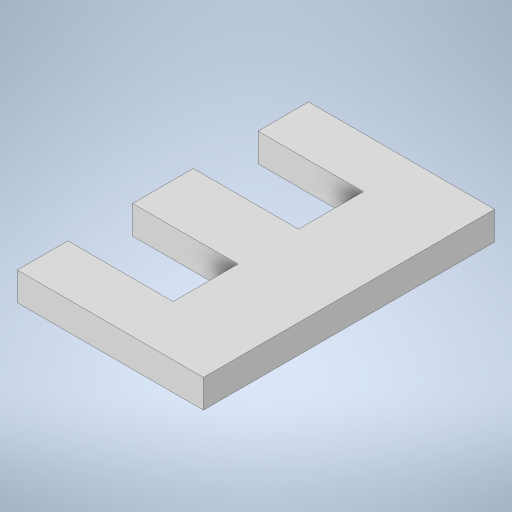
# Autodesk Inventor part: base
Saved by Autodesk Inventor 2024.3 (Build 283343000, 343)
## iProperties
Created: 2024-10-09
Part Number: base
Material: Generic
Document SubType Name: Modeling
Designer: pjcaa
Density: 1 g/cm^3
Appearance: Default
Author: pjcaa
Autodesk Inventor part; units mm, degrees
ref_plane "YZ Plane" through (0, 0, 0) normal (1, 0, 0) x (0, 1, 0)
ref_plane "XZ Plane" through (0, 0, 0) normal (0, 1, 0) x (-1, 0, 0)
ref_plane "XY Plane" through (0, 0, 0) normal (0, 0, 1) x (1, 0, 0)
sketch "Sketch16" plane through (0, 0, 0) normal (0, 0, 1) x (1, 0, 0)
  line L0 (-9, 5.75) -> (9, 5.75)
  line L1 (9, 5.75) -> (9, -5.75)
  line L2 (9, -5.75) -> (-9, -5.75)
  line L3 (-9, -5.75) -> (-9, 5.75)
  line L4 (-9, 5.75) -> (9, -5.75) construction
  line L5 (9, 5.75) -> (-9, -5.75) construction
  point P0 (0, 0)
  dimension "d82" = 18
  dimension "d90" = 11.5
  constraints: 12 end point, 2 midpoint, 2 parallel, 1 horizontal, 1 perpendicular
  measures "d82" distance of L1.end L2.end
  measures "d90" distance of L0.end L1.end
extrude "Extrusion16" add sketch "Sketch16" along normal blind 1.75
sketch "Sketch17" plane through (0, 0, 1.75) normal (0, 0, 1) x (1, 0, 0)
  line L0 (-9, -5.75) -> (9, -5.75) construction
  line L1 (9, -5.75) -> (9, 5.75) construction
  line L2 (9, 5.75) -> (-9, 5.75) construction
  line L3 (-9, 5.75) -> (-9, -5.75) construction
  line L4 (-5.875, 5.75) -> (-1.875, 5.75)
  line L5 (-1.875, 5.75) -> (-1.875, -0.75)
  line L6 (-1.875, -0.75) -> (-5.875, -0.75)
  line L7 (-5.875, -0.75) -> (-5.875, 5.75)
  line L8 (1.875, 5.75) -> (5.875, 5.75)
  line L9 (5.875, 5.75) -> (5.875, -0.75)
  line L10 (5.875, -0.75) -> (1.875, -0.75)
  line L11 (1.875, -0.75) -> (1.875, 5.75)
  line L12 (5.875, -0.75) -> (9, -0.75) construction
  line L13 (1.875, -0.75) -> (-1.875, -0.75) construction
  line L14 (-5.875, -0.75) -> (-9, -0.75) construction
  point P0 (0, 0)
  point P1 (0, -0.75)
  dimension "d85" = 3.75
  dimension "d86" = 4
  dimension "d87" = 6.5
  constraints: 22 end point, 6 point on line, 4 parallel, 3 perpendicular, 2 collinear, 2 horizontal, 1 horizontal alignment, 1 midpoint, 1 vertical alignment
  measures "d85" distance between parallel lines of L11 L5
  measures "d86" distance of L9.end L10.end
  measures "d87" distance of L8.end L9.end
extrude "Extrusion17" cut sketch "Sketch17" against normal through all
body "Solid3"
